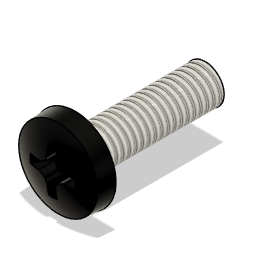
Gearbox v3 (Autodesk Fusion 360 archive; units mm, degrees)
design "Binding Head Screw JIS B 1111 - M3x10 Steel 4.6 Black"
description: Binding Head Screw JIS B 1111 - M3x10
Autodesk Fusion 360 part; units mm, degrees
sketch "Sketch1" plane through (0, 0, 0) normal (0, 1, 0) x (1, 0, 0)
  line L0 (0, -1.9) -> (0, 10)
  line L1 (-3.15, 0) -> (-3.0363, -1.3)
  line L2 (-3.15, 0) -> (-1.399, 0)
  arc A0 (-3.0363, -1.3) -> (0, -1.9) centre (0, 6.0824) ccw
  line L3 (0, 10) -> (-1.5, 10)
  line L4 (-1.5, 10) -> (-1.5, 0.94)
  line L5 (-1.5, 0.94) -> (-1.299, 0.19)
  line L6 (-1.299, 0.19) -> (-1.299, 0.1)
  line L7 (-1.299, 0.1) -> (-1.399, 0.1) construction
  line L8 (-1.399, 0.1) -> (-1.399, 0) construction
  circle A1 centre (-1.399, 0.1) radius 0.1
  dimension "d13" = 5
  dimension "d14" = 6.3
  dimension "d15" = 0.6
  dimension "d17" = 1.3
  dimension "d18" = 3
  dimension "d19" = 10
  dimension "d20" = 9.06
  dimension "d22" = 0.75
  dimension "d23" = 15
  dimension "d24" = 0.1
  dimension "d25" = 0.1
  dimension "d26" = 0.2
  constraint vertical L0
  constraint coincident origin L0
  constraint horizontal L2
  constraint coincident origin L2
  constraint coincident L0 A0.end
  constraint coincident L0 A0.centre
  constraint coincident L0.start A0.end
  constraint perpendicular L0 L3
  constraint perpendicular L3 L4
  constraint vertical L6
  constraint perpendicular L6 L7
  constraint perpendicular L7 L8
  constraint coincident L2.end L8.end
  constraint coincident L7.end L8.start
  measures "d13" angle of L0 L1
  measures "d15" vertical distance of L0.start L1.end
  measures "d17" vertical distance of L1.start L1.end
  measures "d19" distance of L2.end L3
  measures "d20" distance of L3.end L4.end
  measures "d22" vertical distance of L4.end L5.end
  measures "d23" angle of L4 L5
  measures "d24" distance of L7.end L2.end
  measures "d25" distance of L6.end L7.end
  measures "d26" diameter of A1
revolve "Revolve1" add sketch "Sketch1" angle 360 about axis through (0, 0, 1.9) along (0, 0, -1) contours L0 L1 L2 A0 L3 L4 L5 L6 A1 makes body 1
ref_plane "WorkPlane1" through (0, 0, 1.9) normal (0, 0, 1) x (1, 0, 0)
sketch "Sketch2" plane through (0, 0, 1.9) normal (0, 0, 1) x (1, 0, 0)
  line L0 (-1.85, 0) -> (1.85, 0) construction
  line L1 (0, -1.85) -> (0, 1.85) construction
  line L2 (-0.331, 1.85) -> (0.331, 1.85)
  line L3 (0.331, 1.85) -> (0.331, 0.331)
  line L4 (0.331, 0.331) -> (1.85, 0.331)
  line L5 (1.85, 0.331) -> (1.85, -0.331)
  line L6 (1.85, -0.331) -> (0.331, -0.331)
  line L7 (0.331, -0.331) -> (0.331, -1.85)
  line L8 (0.331, -1.85) -> (-0.331, -1.85)
  line L9 (-0.331, -1.85) -> (-0.331, -0.331)
  line L10 (-0.331, -0.331) -> (-1.85, -0.331)
  line L11 (-1.85, -0.331) -> (-1.85, 0.331)
  line L12 (-1.85, 0.331) -> (-0.331, 0.331)
  line L13 (-0.331, 0.331) -> (-0.331, 1.85)
  dimension "d39" = 3.7
  dimension "d40" = 3.7
  dimension "d41" = 0.662
  dimension "d42" = 0.662
  constraint horizontal L0
  constraint vertical L1
  constraint midpoint L0 L1
  constraint midpoint origin L1
  constraint perpendicular L1 L2
  constraint perpendicular L2 L3
  constraint perpendicular L3 L4
  constraint perpendicular L0 L5
  constraint perpendicular L5 L6
  constraint perpendicular L0 L7
  constraint perpendicular L7 L8
  constraint perpendicular L8 L9
  constraint perpendicular L7 L10
  constraint perpendicular L10 L11
  constraint perpendicular L11 L12
  constraint vertical L13
  constraint coincident L9 L12.end
  constraint coincident L3.end L7
  constraint coincident L6 L9.end
  constraint coincident L4 L12.end
  constraint midpoint L0.end L5
  constraint midpoint L1.start L8
  constraint midpoint L1.end L2
  constraint midpoint L0.start L11
  measures "d39" distance of L0.start L0.end
  measures "d40" distance of L1.start L1.end
  measures "d41" distance of L2.start L2.end
  measures "d42" distance of L10.end L11.end
extrude "Extrude1" add sketch "Sketch2" against normal blind 1.53 separate body makes body 2
draft "Draft1" angle -30 neutral plane through (0, 0, 1.9) pull (0, 0, 1) 4 faces at (0.1103, -1.85, 1.39) (-0.1103, 1.85, 1.39) (-1.85, -0.1103, 1.39) (1.85, 0.1103, 1.39) on bodies 2
fillet "Fillet1" radius 0.662 4 edges at (0.331, -0.331, 1.135) (-0.331, -0.331, 1.135) (-0.331, 0.331, 1.135) (0.331, 0.331, 1.135) on bodies 2
combine "Combine1" operation cut target body 1 tool bodies 2
thread "Thread1" "ISO Metric profile 3.0 M3x0.5 6g" major diameter 2.927 minor diameter 2.3555 pitch 0.5 angle 60 resizes the face on face at (-1.4925, -0.1494, -3.96) on bodies 1
equation "adsk_nomdia = 3.00 mm"
equation "adsk_nomlen = 10.00 mm"
equation "adsk_headdia = 6.30 mm"
equation "adsk_bheig = 1.30 mm"
equation "adsk_phildia = 3.70 mm"
equation "adsk_r = 0.10 mm"
equation "adsk_thrlen = 9.06 mm"
equation "adsk_phildepth = 1.53 mm"
equation "adsk_grplen = 0.94 mm"
equation "adsk_runout = 0.75 mm"
equation "adsk_runang = 15.00 deg"
equation "adsk_headang = 5.00 deg"
equation "d13 = adsk_headang"
equation "d14 = adsk_headdia"
equation "d15 = adsk_ovalh"
equation "adsk_ovalh = 0.60 mm"
equation "d17 = adsk_bheig"
equation "d18 = adsk_nomdia"
equation "d19 = adsk_nomlen"
equation "d20 = adsk_thrlen"
equation "d22 = adsk_runout"
equation "d24 = adsk_r"
equation "d25 = adsk_r"
equation "d26 = adsk_r * 2"
equation "d32 = adsk_bheig + adsk_ovalh"
equation "adsk_philwidth = 0.662 mm"
equation "d39 = adsk_phildia"
equation "d40 = adsk_phildia"
equation "d41 = adsk_philwidth"
equation "d42 = adsk_philwidth"
equation "d43 = -adsk_phildepth"
equation "d48 = adsk_philwidth"
